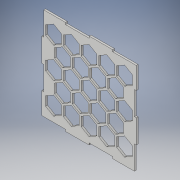
# Autodesk Inventor part: Part1
Saved by Autodesk Inventor 2019 (Build 230136000, 136)
## iProperties
Created: 2019-04-06
Part Number: Part1
Material: Generic
Document SubType Name: Modeling
Designer: Daniel
Density: 1 g/cm^3
Appearance: Default
d0: 14,549 mm
d1: 13,000 ul
d3: 28,200 mm
d4: 13,000 ul
d6: 28,200 mm
d40: 150,000 mm
d41: 150,000 mm
d42: 3,000 mm
d43: 0,00 deg
d44: 3,000 mm
d45: 37,500 mm
d46: 3,000 mm
d47: 37,500 mm
d48: 3,000 mm
d49: 37,500 mm
d50: 3,000 mm
d51: 37,500 mm
d52: 3,000 mm
d53: 37,500 mm
d54: 3,000 mm
d55: 37,500 mm
d56: 3,000 mm
d57: 3,000 mm
d58: 37,500 mm
d59: 3,000 mm
d60: 37,500 mm
d61: 37,500 mm
d62: 37,500 mm
d63: 3,000 mm
d64: 37,500 mm
d65: 3,000 mm
d66: 37,500 mm
d67: 3,000 mm
d68: 62,088 mm
d69: 0,00 deg
Author: Daniel
Autodesk Inventor part; units mm, degrees
(part 1 of 2)
ref_plane "YZ Plane" through (0, 0, 0) normal (1, 0, 0) x (0, 1, 0)
ref_plane "XZ Plane" through (0, 0, 0) normal (0, 1, 0) x (-1, 0, 0)
ref_plane "XY Plane" through (0, 0, 0) normal (0, 0, 1) x (1, 0, 0)
sketch "Sketch1" plane through (0, 0, 0) normal (0, 0, 1) x (1, 0, 0)
  line L0 (0, 0) -> (0, 14.5492)
  line L1 (0, 14.5492) -> (12.6, 7.2746)
  line L2 (12.6, 7.2746) -> (12.6, -7.2746)
  line L3 (12.6, -7.2746) -> (0, -14.5492)
  line L4 (0, -14.5492) -> (-12.6, -7.2746)
  line L5 (-12.6, -7.2746) -> (-12.6, 7.2746)
  line L6 (-12.6, 7.2746) -> (0, 14.5492)
  line L7 (0, 0) -> (-6.3, 10.9119)
  line L8 (0, 0) -> (6.4977, 11.2544)
  line L9 (-14.1, 38.9711) -> (-1.5, 31.6965)
  line L10 (-1.5, 31.6965) -> (-1.5, 17.1473)
  line L11 (-1.5, 17.1473) -> (-14.1, 9.8727)
  line L12 (-14.1, 9.8727) -> (-26.7, 17.1473)
  line L13 (-26.7, 17.1473) -> (-26.7, 31.6965)
  line L14 (-26.7, 31.6965) -> (-14.1, 38.9711)
  line L15 (-28.2, 63.3931) -> (-15.6, 56.1184)
  line L16 (-15.6, 56.1184) -> (-15.6, 41.5692)
  line L17 (-15.6, 41.5692) -> (-28.2, 34.2946)
  line L18 (-28.2, 34.2946) -> (-40.8, 41.5692)
  line L19 (-40.8, 41.5692) -> (-40.8, 56.1184)
  line L20 (-40.8, 56.1184) -> (-28.2, 63.3931)
  line L21 (-42.3, 87.815) -> (-29.7, 80.5404)
  line L22 (-29.7, 80.5404) -> (-29.7, 65.9911)
  line L23 (-29.7, 65.9911) -> (-42.3, 58.7165)
  line L24 (-42.3, 58.7165) -> (-54.9, 65.9911)
  line L25 (-54.9, 65.9911) -> (-54.9, 80.5404)
  line L26 (-54.9, 80.5404) -> (-42.3, 87.815)
  line L27 (-56.4, 112.2369) -> (-43.8, 104.9623)
  line L28 (-43.8, 104.9623) -> (-43.8, 90.4131)
  line L29 (-43.8, 90.4131) -> (-56.4, 83.1384)
  line L30 (-56.4, 83.1384) -> (-69, 90.4131)
  line L31 (-69, 90.4131) -> (-69, 104.9623)
  line L32 (-69, 104.9623) -> (-56.4, 112.2369)
  line L33 (-70.5, 136.6588) -> (-57.9, 129.3842)
  line L34 (-57.9, 129.3842) -> (-57.9, 114.835)
  line L35 (-57.9, 114.835) -> (-70.5, 107.5604)
  line L36 (-70.5, 107.5604) -> (-83.1, 114.835)
  line L37 (-83.1, 114.835) -> (-83.1, 129.3842)
  line L38 (-83.1, 129.3842) -> (-70.5, 136.6588)
  line L39 (-84.6, 161.0807) -> (-72, 153.8061)
  line L40 (-72, 153.8061) -> (-72, 139.2569)
  line L41 (-72, 139.2569) -> (-84.6, 131.9823)
  line L42 (-84.6, 131.9823) -> (-97.2, 139.2569)
  line L43 (-97.2, 139.2569) -> (-97.2, 153.8061)
  line L44 (-97.2, 153.8061) -> (-84.6, 161.0807)
  line L45 (-98.7, 185.5026) -> (-86.1, 178.228)
  line L46 (-86.1, 178.228) -> (-86.1, 163.6788)
  line L47 (-86.1, 163.6788) -> (-98.7, 156.4042)
  line L48 (-98.7, 156.4042) -> (-111.3, 163.6788)
  line L49 (-111.3, 163.6788) -> (-111.3, 178.228)
  line L50 (-111.3, 178.228) -> (-98.7, 185.5026)
  line L51 (-112.8, 209.9246) -> (-100.2, 202.6499)
  line L52 (-100.2, 202.6499) -> (-100.2, 188.1007)
  line L53 (-100.2, 188.1007) -> (-112.8, 180.8261)
  line L54 (-112.8, 180.8261) -> (-125.4, 188.1007)
  line L55 (-125.4, 188.1007) -> (-125.4, 202.6499)
  line L56 (-125.4, 202.6499) -> (-112.8, 209.9246)
  line L57 (-126.9, 234.3465) -> (-114.3, 227.0719)
  line L58 (-114.3, 227.0719) -> (-114.3, 212.5226)
  line L59 (-114.3, 212.5226) -> (-126.9, 205.248)
  line L60 (-126.9, 205.248) -> (-139.5, 212.5226)
  line L61 (-139.5, 212.5226) -> (-139.5, 227.0719)
  line L62 (-139.5, 227.0719) -> (-126.9, 234.3465)
  line L63 (-141, 258.7684) -> (-128.4, 251.4938)
  line L64 (-128.4, 251.4938) -> (-128.4, 236.9446)
  line L65 (-128.4, 236.9446) -> (-141, 229.6699)
  line L66 (-141, 229.6699) -> (-153.6, 236.9446)
  line L67 (-153.6, 236.9446) -> (-153.6, 251.4938)
  line L68 (-153.6, 251.4938) -> (-141, 258.7684)
  line L69 (-155.1, 283.1903) -> (-142.5, 275.9157)
  line L70 (-142.5, 275.9157) -> (-142.5, 261.3665)
  line L71 (-142.5, 261.3665) -> (-155.1, 254.0919)
  line L72 (-155.1, 254.0919) -> (-167.7, 261.3665)
  line L73 (-167.7, 261.3665) -> (-167.7, 275.9157)
  line L74 (-167.7, 275.9157) -> (-155.1, 283.1903)
  line L75 (-169.2, 307.6122) -> (-156.6, 300.3376)
  line L76 (-156.6, 300.3376) -> (-156.6, 285.7884)
  line L77 (-156.6, 285.7884) -> (-169.2, 278.5138)
  line L78 (-169.2, 278.5138) -> (-181.8, 285.7884)
  line L79 (-181.8, 285.7884) -> (-181.8, 300.3376)
  line L80 (-181.8, 300.3376) -> (-169.2, 307.6122)
  line L81 (14.1, 38.9711) -> (26.7, 31.6965)
  line L82 (26.7, 31.6965) -> (26.7, 17.1473)
  line L83 (26.7, 17.1473) -> (14.1, 9.8727)
  line L84 (14.1, 9.8727) -> (1.5, 17.1473)
  line L85 (1.5, 17.1473) -> (1.5, 31.6965)
  line L86 (1.5, 31.6965) -> (14.1, 38.9711)
  line L87 (0, 63.3931) -> (12.6, 56.1184)
  line L88 (12.6, 56.1184) -> (12.6, 41.5692)
  line L89 (12.6, 41.5692) -> (0, 34.2946)
  line L90 (0, 34.2946) -> (-12.6, 41.5692)
  line L91 (-12.6, 41.5692) -> (-12.6, 56.1184)
  line L92 (-12.6, 56.1184) -> (0, 63.3931)
  line L93 (-14.1, 87.815) -> (-1.5, 80.5404)
  line L94 (-1.5, 80.5404) -> (-1.5, 65.9911)
  line L95 (-1.5, 65.9911) -> (-14.1, 58.7165)
  line L96 (-14.1, 58.7165) -> (-26.7, 65.9911)
  line L97 (-26.7, 65.9911) -> (-26.7, 80.5404)
  line L98 (-26.7, 80.5404) -> (-14.1, 87.815)
  line L99 (-28.2, 112.2369) -> (-15.6, 104.9623)
  line L100 (-15.6, 104.9623) -> (-15.6, 90.4131)
  line L101 (-15.6, 90.4131) -> (-28.2, 83.1384)
  line L102 (-28.2, 83.1384) -> (-40.8, 90.4131)
  line L103 (-40.8, 90.4131) -> (-40.8, 104.9623)
  line L104 (-40.8, 104.9623) -> (-28.2, 112.2369)
  line L105 (-42.3, 136.6588) -> (-29.7, 129.3842)
  line L106 (-29.7, 129.3842) -> (-29.7, 114.835)
  line L107 (-29.7, 114.835) -> (-42.3, 107.5604)
  line L108 (-42.3, 107.5604) -> (-54.9, 114.835)
  line L109 (-54.9, 114.835) -> (-54.9, 129.3842)
  line L110 (-54.9, 129.3842) -> (-42.3, 136.6588)
  line L111 (-56.4, 161.0807) -> (-43.8, 153.8061)
  line L112 (-43.8, 153.8061) -> (-43.8, 139.2569)
  line L113 (-43.8, 139.2569) -> (-56.4, 131.9823)
  line L114 (-56.4, 131.9823) -> (-69, 139.2569)
  line L115 (-69, 139.2569) -> (-69, 153.8061)
  line L116 (-69, 153.8061) -> (-56.4, 161.0807)
  line L117 (-70.5, 185.5026) -> (-57.9, 178.228)
  line L118 (-57.9, 178.228) -> (-57.9, 163.6788)
  line L119 (-57.9, 163.6788) -> (-70.5, 156.4042)
  line L120 (-70.5, 156.4042) -> (-83.1, 163.6788)
  line L121 (-83.1, 163.6788) -> (-83.1, 178.228)
  line L122 (-83.1, 178.228) -> (-70.5, 185.5026)
  line L123 (-84.6, 209.9246) -> (-72, 202.6499)
  line L124 (-72, 202.6499) -> (-72, 188.1007)
  line L125 (-72, 188.1007) -> (-84.6, 180.8261)
  line L126 (-84.6, 180.8261) -> (-97.2, 188.1007)
  line L127 (-97.2, 188.1007) -> (-97.2, 202.6499)
  line L128 (-97.2, 202.6499) -> (-84.6, 209.9246)
  line L129 (-98.7, 234.3465) -> (-86.1, 227.0719)
  line L130 (-86.1, 227.0719) -> (-86.1, 212.5226)
  line L131 (-86.1, 212.5226) -> (-98.7, 205.248)
  line L132 (-98.7, 205.248) -> (-111.3, 212.5226)
  line L133 (-111.3, 212.5226) -> (-111.3, 227.0719)
  line L134 (-111.3, 227.0719) -> (-98.7, 234.3465)
  line L135 (-112.8, 258.7684) -> (-100.2, 251.4938)
  line L136 (-100.2, 251.4938) -> (-100.2, 236.9446)
  line L137 (-100.2, 236.9446) -> (-112.8, 229.6699)
  line L138 (-112.8, 229.6699) -> (-125.4, 236.9446)
  line L139 (-125.4, 236.9446) -> (-125.4, 251.4938)
  line L140 (-125.4, 251.4938) -> (-112.8, 258.7684)
  line L141 (-126.9, 283.1903) -> (-114.3, 275.9157)
  line L142 (-114.3, 275.9157) -> (-114.3, 261.3665)
  line L143 (-114.3, 261.3665) -> (-126.9, 254.0919)
  line L144 (-126.9, 254.0919) -> (-139.5, 261.3665)
  line L145 (-139.5, 261.3665) -> (-139.5, 275.9157)
  line L146 (-139.5, 275.9157) -> (-126.9, 283.1903)
  line L147 (-141, 307.6122) -> (-128.4, 300.3376)
  line L148 (-128.4, 300.3376) -> (-128.4, 285.7884)
  line L149 (-128.4, 285.7884) -> (-141, 278.5138)
  line L150 (-141, 278.5138) -> (-153.6, 285.7884)
  line L151 (-153.6, 285.7884) -> (-153.6, 300.3376)
  line L152 (-153.6, 300.3376) -> (-141, 307.6122)
  line L153 (-155.1, 332.0341) -> (-142.5, 324.7595)
  line L154 (-142.5, 324.7595) -> (-142.5, 310.2103)
  line L155 (-142.5, 310.2103) -> (-155.1, 302.9357)
  line L156 (-155.1, 302.9357) -> (-167.7, 310.2103)
  line L157 (-167.7, 310.2103) -> (-167.7, 324.7595)
  line L158 (-167.7, 324.7595) -> (-155.1, 332.0341)
  line L159 (28.2, 63.3931) -> (40.8, 56.1184)
  line L160 (40.8, 56.1184) -> (40.8, 41.5692)
  line L161 (40.8, 41.5692) -> (28.2, 34.2946)
  line L162 (28.2, 34.2946) -> (15.6, 41.5692)
  line L163 (15.6, 41.5692) -> (15.6, 56.1184)
  line L164 (15.6, 56.1184) -> (28.2, 63.3931)
  line L165 (14.1, 87.815) -> (26.7, 80.5404)
  line L166 (26.7, 80.5404) -> (26.7, 65.9911)
  line L167 (26.7, 65.9911) -> (14.1, 58.7165)
  line L168 (14.1, 58.7165) -> (1.5, 65.9911)
  line L169 (1.5, 65.9911) -> (1.5, 80.5404)
  line L170 (1.5, 80.5404) -> (14.1, 87.815)
  line L171 (0, 112.2369) -> (12.6, 104.9623)
  line L172 (12.6, 104.9623) -> (12.6, 90.4131)
  line L173 (12.6, 90.4131) -> (0, 83.1384)
  line L174 (0, 83.1384) -> (-12.6, 90.4131)
  line L175 (-12.6, 90.4131) -> (-12.6, 104.9623)
  line L176 (-12.6, 104.9623) -> (0, 112.2369)
  line L177 (-14.1, 136.6588) -> (-1.5, 129.3842)
  line L178 (-1.5, 129.3842) -> (-1.5, 114.835)
  line L179 (-1.5, 114.835) -> (-14.1, 107.5604)
  line L180 (-14.1, 107.5604) -> (-26.7, 114.835)
  line L181 (-26.7, 114.835) -> (-26.7, 129.3842)
  line L182 (-26.7, 129.3842) -> (-14.1, 136.6588)
  line L183 (-28.2, 161.0807) -> (-15.6, 153.8061)
  line L184 (-15.6, 153.8061) -> (-15.6, 139.2569)
  line L185 (-15.6, 139.2569) -> (-28.2, 131.9823)
  line L186 (-28.2, 131.9823) -> (-40.8, 139.2569)
  line L187 (-40.8, 139.2569) -> (-40.8, 153.8061)
  line L188 (-40.8, 153.8061) -> (-28.2, 161.0807)
  line L189 (-42.3, 185.5026) -> (-29.7, 178.228)
  line L190 (-29.7, 178.228) -> (-29.7, 163.6788)
  line L191 (-29.7, 163.6788) -> (-42.3, 156.4042)
  line L192 (-42.3, 156.4042) -> (-54.9, 163.6788)
  line L193 (-54.9, 163.6788) -> (-54.9, 178.228)
  line L194 (-54.9, 178.228) -> (-42.3, 185.5026)
  line L195 (-56.4, 209.9246) -> (-43.8, 202.6499)
  line L196 (-43.8, 202.6499) -> (-43.8, 188.1007)
  line L197 (-43.8, 188.1007) -> (-56.4, 180.8261)
  line L198 (-56.4, 180.8261) -> (-69, 188.1007)
  line L199 (-69, 188.1007) -> (-69, 202.6499)
  line L200 (-69, 202.6499) -> (-56.4, 209.9246)
  line L201 (-70.5, 234.3465) -> (-57.9, 227.0719)
  line L202 (-57.9, 227.0719) -> (-57.9, 212.5226)
  line L203 (-57.9, 212.5226) -> (-70.5, 205.248)
  line L204 (-70.5, 205.248) -> (-83.1, 212.5226)
  line L205 (-83.1, 212.5226) -> (-83.1, 227.0719)
  line L206 (-83.1, 227.0719) -> (-70.5, 234.3465)
  line L207 (-84.6, 258.7684) -> (-72, 251.4938)
  line L208 (-72, 251.4938) -> (-72, 236.9446)
  line L209 (-72, 236.9446) -> (-84.6, 229.6699)
  line L210 (-84.6, 229.6699) -> (-97.2, 236.9446)
  line L211 (-97.2, 236.9446) -> (-97.2, 251.4938)
  line L212 (-97.2, 251.4938) -> (-84.6, 258.7684)
  line L213 (-98.7, 283.1903) -> (-86.1, 275.9157)
  line L214 (-86.1, 275.9157) -> (-86.1, 261.3665)
  line L215 (-86.1, 261.3665) -> (-98.7, 254.0919)
  line L216 (-98.7, 254.0919) -> (-111.3, 261.3665)
  line L217 (-111.3, 261.3665) -> (-111.3, 275.9157)
  line L218 (-111.3, 275.9157) -> (-98.7, 283.1903)
  line L219 (-112.8, 307.6122) -> (-100.2, 300.3376)
  line L220 (-100.2, 300.3376) -> (-100.2, 285.7884)
  line L221 (-100.2, 285.7884) -> (-112.8, 278.5138)
  line L222 (-112.8, 278.5138) -> (-125.4, 285.7884)
  line L223 (-125.4, 285.7884) -> (-125.4, 300.3376)
  line L224 (-125.4, 300.3376) -> (-112.8, 307.6122)
  line L225 (-126.9, 332.0341) -> (-114.3, 324.7595)
  line L226 (-114.3, 324.7595) -> (-114.3, 310.2103)
  line L227 (-114.3, 310.2103) -> (-126.9, 302.9357)
  line L228 (-126.9, 302.9357) -> (-139.5, 310.2103)
  line L229 (-139.5, 310.2103) -> (-139.5, 324.7595)
  line L230 (-139.5, 324.7595) -> (-126.9, 332.0341)
  line L231 (-141, 356.4561) -> (-128.4, 349.1814)
  line L232 (-128.4, 349.1814) -> (-128.4, 334.6322)
  line L233 (-128.4, 334.6322) -> (-141, 327.3576)
  line L234 (-141, 327.3576) -> (-153.6, 334.6322)
  line L235 (-153.6, 334.6322) -> (-153.6, 349.1814)
  line L236 (-153.6, 349.1814) -> (-141, 356.4561)
  line L237 (42.3, 87.815) -> (54.9, 80.5404)
  line L238 (54.9, 80.5404) -> (54.9, 65.9911)
  line L239 (54.9, 65.9911) -> (42.3, 58.7165)
  line L240 (42.3, 58.7165) -> (29.7, 65.9911)
  line L241 (29.7, 65.9911) -> (29.7, 80.5404)
  line L242 (29.7, 80.5404) -> (42.3, 87.815)
  line L243 (28.2, 112.2369) -> (40.8, 104.9623)
  line L244 (40.8, 104.9623) -> (40.8, 90.4131)
  line L245 (40.8, 90.4131) -> (28.2, 83.1384)
  line L246 (28.2, 83.1384) -> (15.6, 90.4131)
  line L247 (15.6, 90.4131) -> (15.6, 104.9623)
  line L248 (15.6, 104.9623) -> (28.2, 112.2369)
  line L249 (14.1, 136.6588) -> (26.7, 129.3842)
  line L250 (26.7, 129.3842) -> (26.7, 114.835)
  line L251 (26.7, 114.835) -> (14.1, 107.5604)
  line L252 (14.1, 107.5604) -> (1.5, 114.835)
  line L253 (1.5, 114.835) -> (1.5, 129.3842)
  line L254 (1.5, 129.3842) -> (14.1, 136.6588)
  line L255 (0, 161.0807) -> (12.6, 153.8061)
  line L256 (12.6, 153.8061) -> (12.6, 139.2569)
  line L257 (12.6, 139.2569) -> (0, 131.9823)
  line L258 (0, 131.9823) -> (-12.6, 139.2569)
  line L259 (-12.6, 139.2569) -> (-12.6, 153.8061)
  line L260 (-12.6, 153.8061) -> (0, 161.0807)
  line L261 (-14.1, 185.5026) -> (-1.5, 178.228)
  line L262 (-1.5, 178.228) -> (-1.5, 163.6788)
  line L263 (-1.5, 163.6788) -> (-14.1, 156.4042)
  line L264 (-14.1, 156.4042) -> (-26.7, 163.6788)
  line L265 (-26.7, 163.6788) -> (-26.7, 178.228)
  line L266 (-26.7, 178.228) -> (-14.1, 185.5026)
  line L267 (-28.2, 209.9246) -> (-15.6, 202.6499)
  line L268 (-15.6, 202.6499) -> (-15.6, 188.1007)
  line L269 (-15.6, 188.1007) -> (-28.2, 180.8261)
  line L270 (-28.2, 180.8261) -> (-40.8, 188.1007)
  line L271 (-40.8, 188.1007) -> (-40.8, 202.6499)
  line L272 (-40.8, 202.6499) -> (-28.2, 209.9246)
  line L273 (-42.3, 234.3465) -> (-29.7, 227.0719)
  line L274 (-29.7, 227.0719) -> (-29.7, 212.5226)
  line L275 (-29.7, 212.5226) -> (-42.3, 205.248)
  line L276 (-42.3, 205.248) -> (-54.9, 212.5226)
  line L277 (-54.9, 212.5226) -> (-54.9, 227.0719)
  line L278 (-54.9, 227.0719) -> (-42.3, 234.3465)
  line L279 (-56.4, 258.7684) -> (-43.8, 251.4938)
  line L280 (-43.8, 251.4938) -> (-43.8, 236.9446)
  line L281 (-43.8, 236.9446) -> (-56.4, 229.6699)
  line L282 (-56.4, 229.6699) -> (-69, 236.9446)
  line L283 (-69, 236.9446) -> (-69, 251.4938)
  line L284 (-69, 251.4938) -> (-56.4, 258.7684)
  line L285 (-70.5, 283.1903) -> (-57.9, 275.9157)
  line L286 (-57.9, 275.9157) -> (-57.9, 261.3665)
  line L287 (-57.9, 261.3665) -> (-70.5, 254.0919)
  line L288 (-70.5, 254.0919) -> (-83.1, 261.3665)
  line L289 (-83.1, 261.3665) -> (-83.1, 275.9157)
  line L290 (-83.1, 275.9157) -> (-70.5, 283.1903)
  line L291 (-84.6, 307.6122) -> (-72, 300.3376)
  line L292 (-72, 300.3376) -> (-72, 285.7884)
  line L293 (-72, 285.7884) -> (-84.6, 278.5138)
  line L294 (-84.6, 278.5138) -> (-97.2, 285.7884)
  line L295 (-97.2, 285.7884) -> (-97.2, 300.3376)
  line L296 (-97.2, 300.3376) -> (-84.6, 307.6122)
  line L297 (-98.7, 332.0341) -> (-86.1, 324.7595)
  line L298 (-86.1, 324.7595) -> (-86.1, 310.2103)
  line L299 (-86.1, 310.2103) -> (-98.7, 302.9357)
  line L300 (-98.7, 302.9357) -> (-111.3, 310.2103)
  line L301 (-111.3, 310.2103) -> (-111.3, 324.7595)
  line L302 (-111.3, 324.7595) -> (-98.7, 332.0341)
  line L303 (-112.8, 356.4561) -> (-100.2, 349.1814)
  line L304 (-100.2, 349.1814) -> (-100.2, 334.6322)
  line L305 (-100.2, 334.6322) -> (-112.8, 327.3576)
  line L306 (-112.8, 327.3576) -> (-125.4, 334.6322)
  line L307 (-125.4, 334.6322) -> (-125.4, 349.1814)
  line L308 (-125.4, 349.1814) -> (-112.8, 356.4561)
  line L309 (-126.9, 380.878) -> (-114.3, 373.6034)
  line L310 (-114.3, 373.6034) -> (-114.3, 359.0541)
  line L311 (-114.3, 359.0541) -> (-126.9, 351.7795)
  line L312 (-126.9, 351.7795) -> (-139.5, 359.0541)
  line L313 (-139.5, 359.0541) -> (-139.5, 373.6034)
  line L314 (-139.5, 373.6034) -> (-126.9, 380.878)
  line L315 (56.4, 112.2369) -> (69, 104.9623)
  line L316 (69, 104.9623) -> (69, 90.4131)
  line L317 (69, 90.4131) -> (56.4, 83.1384)
  line L318 (56.4, 83.1384) -> (43.8, 90.4131)
  line L319 (43.8, 90.4131) -> (43.8, 104.9623)
  line L320 (43.8, 104.9623) -> (56.4, 112.2369)
  line L321 (42.3, 136.6588) -> (54.9, 129.3842)
  line L322 (54.9, 129.3842) -> (54.9, 114.835)
  line L323 (54.9, 114.835) -> (42.3, 107.5604)
  line L324 (42.3, 107.5604) -> (29.7, 114.835)
  line L325 (29.7, 114.835) -> (29.7, 129.3842)
  line L326 (29.7, 129.3842) -> (42.3, 136.6588)
  line L327 (28.2, 161.0807) -> (40.8, 153.8061)
  line L328 (40.8, 153.8061) -> (40.8, 139.2569)
  line L329 (40.8, 139.2569) -> (28.2, 131.9823)
  line L330 (28.2, 131.9823) -> (15.6, 139.2569)
  line L331 (15.6, 139.2569) -> (15.6, 153.8061)
  line L332 (15.6, 153.8061) -> (28.2, 161.0807)
  line L333 (14.1, 185.5026) -> (26.7, 178.228)
  line L334 (26.7, 178.228) -> (26.7, 163.6788)
  line L335 (26.7, 163.6788) -> (14.1, 156.4042)
  line L336 (14.1, 156.4042) -> (1.5, 163.6788)
  line L337 (1.5, 163.6788) -> (1.5, 178.228)
  line L338 (1.5, 178.228) -> (14.1, 185.5026)
  line L339 (0, 209.9246) -> (12.6, 202.6499)
  line L340 (12.6, 202.6499) -> (12.6, 188.1007)
  line L341 (12.6, 188.1007) -> (0, 180.8261)
  line L342 (0, 180.8261) -> (-12.6, 188.1007)
  line L343 (-12.6, 188.1007) -> (-12.6, 202.6499)
  line L344 (-12.6, 202.6499) -> (0, 209.9246)
  line L345 (-14.1, 234.3465) -> (-1.5, 227.0719)
  line L346 (-1.5, 227.0719) -> (-1.5, 212.5226)
  line L347 (-1.5, 212.5226) -> (-14.1, 205.248)
  line L348 (-14.1, 205.248) -> (-26.7, 212.5226)
  line L349 (-26.7, 212.5226) -> (-26.7, 227.0719)
  line L350 (-26.7, 227.0719) -> (-14.1, 234.3465)
  line L351 (-28.2, 258.7684) -> (-15.6, 251.4938)
  line L352 (-15.6, 251.4938) -> (-15.6, 236.9446)
  line L353 (-15.6, 236.9446) -> (-28.2, 229.6699)
  line L354 (-28.2, 229.6699) -> (-40.8, 236.9446)
  line L355 (-40.8, 236.9446) -> (-40.8, 251.4938)
  line L356 (-40.8, 251.4938) -> (-28.2, 258.7684)
  line L357 (-42.3, 283.1903) -> (-29.7, 275.9157)
  line L358 (-29.7, 275.9157) -> (-29.7, 261.3665)
  line L359 (-29.7, 261.3665) -> (-42.3, 254.0919)
  line L360 (-42.3, 254.0919) -> (-54.9, 261.3665)
  line L361 (-54.9, 261.3665) -> (-54.9, 275.9157)
  line L362 (-54.9, 275.9157) -> (-42.3, 283.1903)
  line L363 (-56.4, 307.6122) -> (-43.8, 300.3376)
  line L364 (-43.8, 300.3376) -> (-43.8, 285.7884)
  line L365 (-43.8, 285.7884) -> (-56.4, 278.5138)
  line L366 (-56.4, 278.5138) -> (-69, 285.7884)
  line L367 (-69, 285.7884) -> (-69, 300.3376)
  line L368 (-69, 300.3376) -> (-56.4, 307.6122)
  line L369 (-70.5, 332.0341) -> (-57.9, 324.7595)
  line L370 (-57.9, 324.7595) -> (-57.9, 310.2103)
  line L371 (-57.9, 310.2103) -> (-70.5, 302.9357)
  line L372 (-70.5, 302.9357) -> (-83.1, 310.2103)
  line L373 (-83.1, 310.2103) -> (-83.1, 324.7595)
  line L374 (-83.1, 324.7595) -> (-70.5, 332.0341)
  line L375 (-84.6, 356.4561) -> (-72, 349.1814)
  line L376 (-72, 349.1814) -> (-72, 334.6322)
  line L377 (-72, 334.6322) -> (-84.6, 327.3576)
  line L378 (-84.6, 327.3576) -> (-97.2, 334.6322)
  line L379 (-97.2, 334.6322) -> (-97.2, 349.1814)
  line L380 (-97.2, 349.1814) -> (-84.6, 356.4561)
  line L381 (-98.7, 380.878) -> (-86.1, 373.6034)
  line L382 (-86.1, 373.6034) -> (-86.1, 359.0541)
  line L383 (-86.1, 359.0541) -> (-98.7, 351.7795)
  line L384 (-98.7, 351.7795) -> (-111.3, 359.0541)
  line L385 (-111.3, 359.0541) -> (-111.3, 373.6034)
  line L386 (-111.3, 373.6034) -> (-98.7, 380.878)
  line L387 (-112.8, 405.2999) -> (-100.2, 398.0253)
  line L388 (-100.2, 398.0253) -> (-100.2, 383.476)
  line L389 (-100.2, 383.476) -> (-112.8, 376.2014)
  line L390 (-112.8, 376.2014) -> (-125.4, 383.476)
  line L391 (-125.4, 383.476) -> (-125.4, 398.0253)
  line L392 (-125.4, 398.0253) -> (-112.8, 405.2999)
  line L393 (70.5, 136.6588) -> (83.1, 129.3842)
  line L394 (83.1, 129.3842) -> (83.1, 114.835)
  line L395 (83.1, 114.835) -> (70.5, 107.5604)
  line L396 (70.5, 107.5604) -> (57.9, 114.835)
  line L397 (57.9, 114.835) -> (57.9, 129.3842)
  line L398 (57.9, 129.3842) -> (70.5, 136.6588)
  line L399 (56.4, 161.0807) -> (69, 153.8061)
  line L400 (69, 153.8061) -> (69, 139.2569)
  line L401 (69, 139.2569) -> (56.4, 131.9823)
  line L402 (56.4, 131.9823) -> (43.8, 139.2569)
  line L403 (43.8, 139.2569) -> (43.8, 153.8061)
  line L404 (43.8, 153.8061) -> (56.4, 161.0807)
  line L405 (42.3, 185.5026) -> (54.9, 178.228)
  line L406 (54.9, 178.228) -> (54.9, 163.6788)
  line L407 (54.9, 163.6788) -> (42.3, 156.4042)
  line L408 (42.3, 156.4042) -> (29.7, 163.6788)
  line L409 (29.7, 163.6788) -> (29.7, 178.228)
  line L410 (29.7, 178.228) -> (42.3, 185.5026)
  line L411 (28.2, 209.9246) -> (40.8, 202.6499)
  line L412 (40.8, 202.6499) -> (40.8, 188.1007)
  line L413 (40.8, 188.1007) -> (28.2, 180.8261)
  line L414 (28.2, 180.8261) -> (15.6, 188.1007)
  line L415 (15.6, 188.1007) -> (15.6, 202.6499)
  line L416 (15.6, 202.6499) -> (28.2, 209.9246)
  line L417 (14.1, 234.3465) -> (26.7, 227.0719)
  line L418 (26.7, 227.0719) -> (26.7, 212.5226)
  line L419 (26.7, 212.5226) -> (14.1, 205.248)
  line L420 (14.1, 205.248) -> (1.5, 212.5226)
  line L421 (1.5, 212.5226) -> (1.5, 227.0719)
  line L422 (1.5, 227.0719) -> (14.1, 234.3465)
  line L423 (0, 258.7684) -> (12.6, 251.4938)
  line L424 (12.6, 251.4938) -> (12.6, 236.9446)
  line L425 (12.6, 236.9446) -> (0, 229.6699)
  line L426 (0, 229.6699) -> (-12.6, 236.9446)
  line L427 (-12.6, 236.9446) -> (-12.6, 251.4938)
  line L428 (-12.6, 251.4938) -> (0, 258.7684)
  line L429 (-14.1, 283.1903) -> (-1.5, 275.9157)
  line L430 (-1.5, 275.9157) -> (-1.5, 261.3665)
  line L431 (-1.5, 261.3665) -> (-14.1, 254.0919)
  line L432 (-14.1, 254.0919) -> (-26.7, 261.3665)
  line L433 (-26.7, 261.3665) -> (-26.7, 275.9157)
  line L434 (-26.7, 275.9157) -> (-14.1, 283.1903)
  line L435 (-28.2, 307.6122) -> (-15.6, 300.3376)
  line L436 (-15.6, 300.3376) -> (-15.6, 285.7884)
  line L437 (-15.6, 285.7884) -> (-28.2, 278.5138)
  line L438 (-28.2, 278.5138) -> (-40.8, 285.7884)
  line L439 (-40.8, 285.7884) -> (-40.8, 300.3376)
  line L440 (-40.8, 300.3376) -> (-28.2, 307.6122)
  line L441 (-42.3, 332.0341) -> (-29.7, 324.7595)
  line L442 (-29.7, 324.7595) -> (-29.7, 310.2103)
  line L443 (-29.7, 310.2103) -> (-42.3, 302.9357)
  line L444 (-42.3, 302.9357) -> (-54.9, 310.2103)
  line L445 (-54.9, 310.2103) -> (-54.9, 324.7595)
  line L446 (-54.9, 324.7595) -> (-42.3, 332.0341)
  line L447 (-56.4, 356.4561) -> (-43.8, 349.1814)
  line L448 (-43.8, 349.1814) -> (-43.8, 334.6322)
  line L449 (-43.8, 334.6322) -> (-56.4, 327.3576)
  line L450 (-56.4, 327.3576) -> (-69, 334.6322)
  line L451 (-69, 334.6322) -> (-69, 349.1814)
  line L452 (-69, 349.1814) -> (-56.4, 356.4561)
  line L453 (-70.5, 380.878) -> (-57.9, 373.6034)
  line L454 (-57.9, 373.6034) -> (-57.9, 359.0541)
  line L455 (-57.9, 359.0541) -> (-70.5, 351.7795)
  line L456 (-70.5, 351.7795) -> (-83.1, 359.0541)
  line L457 (-83.1, 359.0541) -> (-83.1, 373.6034)
  line L458 (-83.1, 373.6034) -> (-70.5, 380.878)
  line L459 (-84.6, 405.2999) -> (-72, 398.0253)
  line L460 (-72, 398.0253) -> (-72, 383.476)
  line L461 (-72, 383.476) -> (-84.6, 376.2014)
  line L462 (-84.6, 376.2014) -> (-97.2, 383.476)
  line L463 (-97.2, 383.476) -> (-97.2, 398.0253)
  line L464 (-97.2, 398.0253) -> (-84.6, 405.2999)
  line L465 (-98.7, 429.7218) -> (-86.1, 422.4472)
  line L466 (-86.1, 422.4472) -> (-86.1, 407.898)
  line L467 (-86.1, 407.898) -> (-98.7, 400.6234)
  line L468 (-98.7, 400.6234) -> (-111.3, 407.898)
  line L469 (-111.3, 407.898) -> (-111.3, 422.4472)
  line L470 (-111.3, 422.4472) -> (-98.7, 429.7218)
  line L471 (84.6, 161.0807) -> (97.2, 153.8061)
  line L472 (97.2, 153.8061) -> (97.2, 139.2569)
  line L473 (97.2, 139.2569) -> (84.6, 131.9823)
  line L474 (84.6, 131.9823) -> (72, 139.2569)
  line L475 (72, 139.2569) -> (72, 153.8061)
  line L476 (72, 153.8061) -> (84.6, 161.0807)
  line L477 (70.5, 185.5026) -> (83.1, 178.228)
  line L478 (83.1, 178.228) -> (83.1, 163.6788)
  line L479 (83.1, 163.6788) -> (70.5, 156.4042)
  line L480 (70.5, 156.4042) -> (57.9, 163.6788)
  line L481 (57.9, 163.6788) -> (57.9, 178.228)
  line L482 (57.9, 178.228) -> (70.5, 185.5026)
  line L483 (56.4, 209.9246) -> (69, 202.6499)
  line L484 (69, 202.6499) -> (69, 188.1007)
  line L485 (69, 188.1007) -> (56.4, 180.8261)
  line L486 (56.4, 180.8261) -> (43.8, 188.1007)
  line L487 (43.8, 188.1007) -> (43.8, 202.6499)
  line L488 (43.8, 202.6499) -> (56.4, 209.9246)
  line L489 (42.3, 234.3465) -> (54.9, 227.0719)
  line L490 (54.9, 227.0719) -> (54.9, 212.5226)
  line L491 (54.9, 212.5226) -> (42.3, 205.248)
  line L492 (42.3, 205.248) -> (29.7, 212.5226)
  line L493 (29.7, 212.5226) -> (29.7, 227.0719)
  line L494 (29.7, 227.0719) -> (42.3, 234.3465)
  line L495 (28.2, 258.7684) -> (40.8, 251.4938)
  line L496 (40.8, 251.4938) -> (40.8, 236.9446)
  line L497 (40.8, 236.9446) -> (28.2, 229.6699)
  line L498 (28.2, 229.6699) -> (15.6, 236.9446)
  line L499 (15.6, 236.9446) -> (15.6, 251.4938)
  line L500 (15.6, 251.4938) -> (28.2, 258.7684)
  line L501 (14.1, 283.1903) -> (26.7, 275.9157)
  line L502 (26.7, 275.9157) -> (26.7, 261.3665)
  line L503 (26.7, 261.3665) -> (14.1, 254.0919)
  line L504 (14.1, 254.0919) -> (1.5, 261.3665)
  line L505 (1.5, 261.3665) -> (1.5, 275.9157)
  line L506 (1.5, 275.9157) -> (14.1, 283.1903)
  line L507 (0, 307.6122) -> (12.6, 300.3376)
  line L508 (12.6, 300.3376) -> (12.6, 285.7884)
  line L509 (12.6, 285.7884) -> (0, 278.5138)
  line L510 (0, 278.5138) -> (-12.6, 285.7884)
  line L511 (-12.6, 285.7884) -> (-12.6, 300.3376)
  line L512 (-12.6, 300.3376) -> (0, 307.6122)
  line L513 (-14.1, 332.0341) -> (-1.5, 324.7595)
  line L514 (-1.5, 324.7595) -> (-1.5, 310.2103)
  line L515 (-1.5, 310.2103) -> (-14.1, 302.9357)
  line L516 (-14.1, 302.9357) -> (-26.7, 310.2103)
  line L517 (-26.7, 310.2103) -> (-26.7, 324.7595)
  line L518 (-26.7, 324.7595) -> (-14.1, 332.0341)
  line L519 (-28.2, 356.4561) -> (-15.6, 349.1814)
  line L520 (-15.6, 349.1814) -> (-15.6, 334.6322)
  line L521 (-15.6, 334.6322) -> (-28.2, 327.3576)
  line L522 (-28.2, 327.3576) -> (-40.8, 334.6322)
  line L523 (-40.8, 334.6322) -> (-40.8, 349.1814)
  line L524 (-40.8, 349.1814) -> (-28.2, 356.4561)
  line L525 (-42.3, 380.878) -> (-29.7, 373.6034)
  line L526 (-29.7, 373.6034) -> (-29.7, 359.0541)
  line L527 (-29.7, 359.0541) -> (-42.3, 351.7795)
  line L528 (-42.3, 351.7795) -> (-54.9, 359.0541)
  line L529 (-54.9, 359.0541) -> (-54.9, 373.6034)
  line L530 (-54.9, 373.6034) -> (-42.3, 380.878)
  line L531 (-56.4, 405.2999) -> (-43.8, 398.0253)
  line L532 (-43.8, 398.0253) -> (-43.8, 383.476)
  line L533 (-43.8, 383.476) -> (-56.4, 376.2014)
  line L534 (-56.4, 376.2014) -> (-69, 383.476)
  line L535 (-69, 383.476) -> (-69, 398.0253)
  line L536 (-69, 398.0253) -> (-56.4, 405.2999)
  line L537 (-70.5, 429.7218) -> (-57.9, 422.4472)
  line L538 (-57.9, 422.4472) -> (-57.9, 407.898)
  line L539 (-57.9, 407.898) -> (-70.5, 400.6234)
  line L540 (-70.5, 400.6234) -> (-83.1, 407.898)
  line L541 (-83.1, 407.898) -> (-83.1, 422.4472)
  line L542 (-83.1, 422.4472) -> (-70.5, 429.7218)
  line L543 (-84.6, 454.1437) -> (-72, 446.8691)
  line L544 (-72, 446.8691) -> (-72, 432.3199)
  line L545 (-72, 432.3199) -> (-84.6, 425.0453)
  line L546 (-84.6, 425.0453) -> (-97.2, 432.3199)
  line L547 (-97.2, 432.3199) -> (-97.2, 446.8691)
  line L548 (-97.2, 446.8691) -> (-84.6, 454.1437)
  line L549 (98.7, 185.5026) -> (111.3, 178.228)
  line L550 (111.3, 178.228) -> (111.3, 163.6788)
  line L551 (111.3, 163.6788) -> (98.7, 156.4042)
  line L552 (98.7, 156.4042) -> (86.1, 163.6788)
  line L553 (86.1, 163.6788) -> (86.1, 178.228)
  line L554 (86.1, 178.228) -> (98.7, 185.5026)
  line L555 (84.6, 209.9246) -> (97.2, 202.6499)
  line L556 (97.2, 202.6499) -> (97.2, 188.1007)
  line L557 (97.2, 188.1007) -> (84.6, 180.8261)
  line L558 (84.6, 180.8261) -> (72, 188.1007)
  line L559 (72, 188.1007) -> (72, 202.6499)
  line L560 (72, 202.6499) -> (84.6, 209.9246)
  line L561 (70.5, 234.3465) -> (83.1, 227.0719)
  line L562 (83.1, 227.0719) -> (83.1, 212.5226)
  line L563 (83.1, 212.5226) -> (70.5, 205.248)
  line L564 (70.5, 205.248) -> (57.9, 212.5226)
  line L565 (57.9, 212.5226) -> (57.9, 227.0719)
  line L566 (57.9, 227.0719) -> (70.5, 234.3465)
  line L567 (56.4, 258.7684) -> (69, 251.4938)
  line L568 (69, 251.4938) -> (69, 236.9446)
  line L569 (69, 236.9446) -> (56.4, 229.6699)
  line L570 (56.4, 229.6699) -> (43.8, 236.9446)
  line L571 (43.8, 236.9446) -> (43.8, 251.4938)
  line L572 (43.8, 251.4938) -> (56.4, 258.7684)
  line L573 (42.3, 283.1903) -> (54.9, 275.9157)
  line L574 (54.9, 275.9157) -> (54.9, 261.3665)
  line L575 (54.9, 261.3665) -> (42.3, 254.0919)
  line L576 (42.3, 254.0919) -> (29.7, 261.3665)
  line L577 (29.7, 261.3665) -> (29.7, 275.9157)
  line L578 (29.7, 275.9157) -> (42.3, 283.1903)
  line L579 (28.2, 307.6122) -> (40.8, 300.3376)
  line L580 (40.8, 300.3376) -> (40.8, 285.7884)
  line L581 (40.8, 285.7884) -> (28.2, 278.5138)
  line L582 (28.2, 278.5138) -> (15.6, 285.7884)
  line L583 (15.6, 285.7884) -> (15.6, 300.3376)
  line L584 (15.6, 300.3376) -> (28.2, 307.6122)
  line L585 (14.1, 332.0341) -> (26.7, 324.7595)
  line L586 (26.7, 324.7595) -> (26.7, 310.2103)
  line L587 (26.7, 310.2103) -> (14.1, 302.9357)
  line L588 (14.1, 302.9357) -> (1.5, 310.2103)
  line L589 (1.5, 310.2103) -> (1.5, 324.7595)
  line L590 (1.5, 324.7595) -> (14.1, 332.0341)
  line L591 (0, 356.4561) -> (12.6, 349.1814)
  line L592 (12.6, 349.1814) -> (12.6, 334.6322)
  line L593 (12.6, 334.6322) -> (0, 327.3576)
  line L594 (0, 327.3576) -> (-12.6, 334.6322)
  line L595 (-12.6, 334.6322) -> (-12.6, 349.1814)
  line L596 (-12.6, 349.1814) -> (0, 356.4561)
  line L597 (-14.1, 380.878) -> (-1.5, 373.6034)
  line L598 (-1.5, 373.6034) -> (-1.5, 359.0541)
  line L599 (-1.5, 359.0541) -> (-14.1, 351.7795)
  line L600 (-14.1, 351.7795) -> (-26.7, 359.0541)
  line L601 (-26.7, 359.0541) -> (-26.7, 373.6034)
  line L602 (-26.7, 373.6034) -> (-14.1, 380.878)
  line L603 (-28.2, 405.2999) -> (-15.6, 398.0253)
  line L604 (-15.6, 398.0253) -> (-15.6, 383.476)
  line L605 (-15.6, 383.476) -> (-28.2, 376.2014)
  line L606 (-28.2, 376.2014) -> (-40.8, 383.476)
  line L607 (-40.8, 383.476) -> (-40.8, 398.0253)
  line L608 (-40.8, 398.0253) -> (-28.2, 405.2999)
  line L609 (-42.3, 429.7218) -> (-29.7, 422.4472)
  line L610 (-29.7, 422.4472) -> (-29.7, 407.898)
  line L611 (-29.7, 407.898) -> (-42.3, 400.6234)
  line L612 (-42.3, 400.6234) -> (-54.9, 407.898)
  line L613 (-54.9, 407.898) -> (-54.9, 422.4472)
  line L614 (-54.9, 422.4472) -> (-42.3, 429.7218)
  line L615 (-56.4, 454.1437) -> (-43.8, 446.8691)
  line L616 (-43.8, 446.8691) -> (-43.8, 432.3199)
  line L617 (-43.8, 432.3199) -> (-56.4, 425.0453)
  line L618 (-56.4, 425.0453) -> (-69, 432.3199)
  line L619 (-69, 432.3199) -> (-69, 446.8691)
  line L620 (-69, 446.8691) -> (-56.4, 454.1437)
  line L621 (-70.5, 478.5656) -> (-57.9, 471.291)
  line L622 (-57.9, 471.291) -> (-57.9, 456.7418)
  line L623 (-57.9, 456.7418) -> (-70.5, 449.4672)
  line L624 (-70.5, 449.4672) -> (-83.1, 456.7418)
  line L625 (-83.1, 456.7418) -> (-83.1, 471.291)
  line L626 (-83.1, 471.291) -> (-70.5, 478.5656)
  line L627 (112.8, 209.9246) -> (125.4, 202.6499)
  line L628 (125.4, 202.6499) -> (125.4, 188.1007)
  line L629 (125.4, 188.1007) -> (112.8, 180.8261)
  line L630 (112.8, 180.8261) -> (100.2, 188.1007)
  line L631 (100.2, 188.1007) -> (100.2, 202.6499)
  line L632 (100.2, 202.6499) -> (112.8, 209.9246)
  line L633 (98.7, 234.3465) -> (111.3, 227.0719)
  line L634 (111.3, 227.0719) -> (111.3, 212.5226)
  line L635 (111.3, 212.5226) -> (98.7, 205.248)
  line L636 (98.7, 205.248) -> (86.1, 212.5226)
  line L637 (86.1, 212.5226) -> (86.1, 227.0719)
  line L638 (86.1, 227.0719) -> (98.7, 234.3465)
  line L639 (84.6, 258.7684) -> (97.2, 251.4938)
  line L640 (97.2, 251.4938) -> (97.2, 236.9446)
  line L641 (97.2, 236.9446) -> (84.6, 229.6699)
  line L642 (84.6, 229.6699) -> (72, 236.9446)
  line L643 (72, 236.9446) -> (72, 251.4938)
  line L644 (72, 251.4938) -> (84.6, 258.7684)
  line L645 (70.5, 283.1903) -> (83.1, 275.9157)
  line L646 (83.1, 275.9157) -> (83.1, 261.3665)
  line L647 (83.1, 261.3665) -> (70.5, 254.0919)
  line L648 (70.5, 254.0919) -> (57.9, 261.3665)
  line L649 (57.9, 261.3665) -> (57.9, 275.9157)
  line L650 (57.9, 275.9157) -> (70.5, 283.1903)
  line L651 (56.4, 307.6122) -> (69, 300.3376)
  line L652 (69, 300.3376) -> (69, 285.7884)
  line L653 (69, 285.7884) -> (56.4, 278.5138)
  line L654 (56.4, 278.5138) -> (43.8, 285.7884)
  line L655 (43.8, 285.7884) -> (43.8, 300.3376)
  line L656 (43.8, 300.3376) -> (56.4, 307.6122)
  line L657 (42.3, 332.0341) -> (54.9, 324.7595)
  line L658 (54.9, 324.7595) -> (54.9, 310.2103)
  line L659 (54.9, 310.2103) -> (42.3, 302.9357)
  line L660 (42.3, 302.9357) -> (29.7, 310.2103)
  line L661 (29.7, 310.2103) -> (29.7, 324.7595)
  line L662 (29.7, 324.7595) -> (42.3, 332.0341)
  line L663 (28.2, 356.4561) -> (40.8, 349.1814)
  line L664 (40.8, 349.1814) -> (40.8, 334.6322)
  line L665 (40.8, 334.6322) -> (28.2, 327.3576)
  line L666 (28.2, 327.3576) -> (15.6, 334.6322)
  line L667 (15.6, 334.6322) -> (15.6, 349.1814)
  line L668 (15.6, 349.1814) -> (28.2, 356.4561)
  line L669 (14.1, 380.878) -> (26.7, 373.6034)
  line L670 (26.7, 373.6034) -> (26.7, 359.0541)
  line L671 (26.7, 359.0541) -> (14.1, 351.7795)
  line L672 (14.1, 351.7795) -> (1.5, 359.0541)
  line L673 (1.5, 359.0541) -> (1.5, 373.6034)
  line L674 (1.5, 373.6034) -> (14.1, 380.878)
  line L675 (0, 405.2999) -> (12.6, 398.0253)
  line L676 (12.6, 398.0253) -> (12.6, 383.476)
  line L677 (12.6, 383.476) -> (0, 376.2014)
  line L678 (0, 376.2014) -> (-12.6, 383.476)
  line L679 (-12.6, 383.476) -> (-12.6, 398.0253)
  line L680 (-12.6, 398.0253) -> (0, 405.2999)
  line L681 (-14.1, 429.7218) -> (-1.5, 422.4472)
  line L682 (-1.5, 422.4472) -> (-1.5, 407.898)
  line L683 (-1.5, 407.898) -> (-14.1, 400.6234)
  line L684 (-14.1, 400.6234) -> (-26.7, 407.898)
  line L685 (-26.7, 407.898) -> (-26.7, 422.4472)
  line L686 (-26.7, 422.4472) -> (-14.1, 429.7218)
  line L687 (-28.2, 454.1437) -> (-15.6, 446.8691)
  line L688 (-15.6, 446.8691) -> (-15.6, 432.3199)
  line L689 (-15.6, 432.3199) -> (-28.2, 425.0453)
  line L690 (-28.2, 425.0453) -> (-40.8, 432.3199)
  line L691 (-40.8, 432.3199) -> (-40.8, 446.8691)
  line L692 (-40.8, 446.8691) -> (-28.2, 454.1437)
  line L693 (-42.3, 478.5656) -> (-29.7, 471.291)
  line L694 (-29.7, 471.291) -> (-29.7, 456.7418)
  line L695 (-29.7, 456.7418) -> (-42.3, 449.4672)
  line L696 (-42.3, 449.4672) -> (-54.9, 456.7418)
  line L697 (-54.9, 456.7418) -> (-54.9, 471.291)
  line L698 (-54.9, 471.291) -> (-42.3, 478.5656)
  line L699 (-56.4, 502.9876) -> (-43.8, 495.7129)
  line L700 (-43.8, 495.7129) -> (-43.8, 481.1637)
  line L701 (-43.8, 481.1637) -> (-56.4, 473.8891)
  line L702 (-56.4, 473.8891) -> (-69, 481.1637)
  line L703 (-69, 481.1637) -> (-69, 495.7129)
  line L704 (-69, 495.7129) -> (-56.4, 502.9876)
  line L705 (126.9, 234.3465) -> (139.5, 227.0719)
  line L706 (139.5, 227.0719) -> (139.5, 212.5226)
  line L707 (139.5, 212.5226) -> (126.9, 205.248)
  line L708 (126.9, 205.248) -> (114.3, 212.5226)
  line L709 (114.3, 212.5226) -> (114.3, 227.0719)
  line L710 (114.3, 227.0719) -> (126.9, 234.3465)
  line L711 (112.8, 258.7684) -> (125.4, 251.4938)
  line L712 (125.4, 251.4938) -> (125.4, 236.9446)
  line L713 (125.4, 236.9446) -> (112.8, 229.6699)
  line L714 (112.8, 229.6699) -> (100.2, 236.9446)
  line L715 (100.2, 236.9446) -> (100.2, 251.4938)
  line L716 (100.2, 251.4938) -> (112.8, 258.7684)
  line L717 (98.7, 283.1903) -> (111.3, 275.9157)
  line L718 (111.3, 275.9157) -> (111.3, 261.3665)
  line L719 (111.3, 261.3665) -> (98.7, 254.0919)
  line L720 (98.7, 254.0919) -> (86.1, 261.3665)
  line L721 (86.1, 261.3665) -> (86.1, 275.9157)
  line L722 (86.1, 275.9157) -> (98.7, 283.1903)
  line L723 (84.6, 307.6122) -> (97.2, 300.3376)
  line L724 (97.2, 300.3376) -> (97.2, 285.7884)
  line L725 (97.2, 285.7884) -> (84.6, 278.5138)
  line L726 (84.6, 278.5138) -> (72, 285.7884)
  line L727 (72, 285.7884) -> (72, 300.3376)
  line L728 (72, 300.3376) -> (84.6, 307.6122)
  line L729 (70.5, 332.0341) -> (83.1, 324.7595)
  line L730 (83.1, 324.7595) -> (83.1, 310.2103)
  line L731 (83.1, 310.2103) -> (70.5, 302.9357)
  line L732 (70.5, 302.9357) -> (57.9, 310.2103)
  line L733 (57.9, 310.2103) -> (57.9, 324.7595)
  line L734 (57.9, 324.7595) -> (70.5, 332.0341)
  line L735 (56.4, 356.4561) -> (69, 349.1814)
  line L736 (69, 349.1814) -> (69, 334.6322)
  line L737 (69, 334.6322) -> (56.4, 327.3576)
  line L738 (56.4, 327.3576) -> (43.8, 334.6322)
  line L739 (43.8, 334.6322) -> (43.8, 349.1814)
  line L740 (43.8, 349.1814) -> (56.4, 356.4561)
  line L741 (42.3, 380.878) -> (54.9, 373.6034)
  line L742 (54.9, 373.6034) -> (54.9, 359.0541)
  line L743 (54.9, 359.0541) -> (42.3, 351.7795)
  line L744 (42.3, 351.7795) -> (29.7, 359.0541)
  line L745 (29.7, 359.0541) -> (29.7, 373.6034)
  line L746 (29.7, 373.6034) -> (42.3, 380.878)
  line L747 (28.2, 405.2999) -> (40.8, 398.0253)
  line L748 (40.8, 398.0253) -> (40.8, 383.476)
  line L749 (40.8, 383.476) -> (28.2, 376.2014)
  line L750 (28.2, 376.2014) -> (15.6, 383.476)
  line L751 (15.6, 383.476) -> (15.6, 398.0253)
  line L752 (15.6, 398.0253) -> (28.2, 405.2999)
  line L753 (14.1, 429.7218) -> (26.7, 422.4472)
  line L754 (26.7, 422.4472) -> (26.7, 407.898)
  line L755 (26.7, 407.898) -> (14.1, 400.6234)
  line L756 (14.1, 400.6234) -> (1.5, 407.898)
  line L757 (1.5, 407.898) -> (1.5, 422.4472)
  line L758 (1.5, 422.4472) -> (14.1, 429.7218)
  line L759 (0, 454.1437) -> (12.6, 446.8691)
  line L760 (12.6, 446.8691) -> (12.6, 432.3199)
  line L761 (12.6, 432.3199) -> (0, 425.0453)
  line L762 (0, 425.0453) -> (-12.6, 432.3199)
  line L763 (-12.6, 432.3199) -> (-12.6, 446.8691)
  line L764 (-12.6, 446.8691) -> (0, 454.1437)
  line L765 (-14.1, 478.5656) -> (-1.5, 471.291)
  line L766 (-1.5, 471.291) -> (-1.5, 456.7418)
  line L767 (-1.5, 456.7418) -> (-14.1, 449.4672)
  line L768 (-14.1, 449.4672) -> (-26.7, 456.7418)
  line L769 (-26.7, 456.7418) -> (-26.7, 471.291)
  line L770 (-26.7, 471.291) -> (-14.1, 478.5656)
  line L771 (-28.2, 502.9876) -> (-15.6, 495.7129)
  line L772 (-15.6, 495.7129) -> (-15.6, 481.1637)
  line L773 (-15.6, 481.1637) -> (-28.2, 473.8891)
  line L774 (-28.2, 473.8891) -> (-40.8, 481.1637)
  line L775 (-40.8, 481.1637) -> (-40.8, 495.7129)
  line L776 (-40.8, 495.7129) -> (-28.2, 502.9876)
  line L777 (-42.3, 527.4095) -> (-29.7, 520.1349)
  line L778 (-29.7, 520.1349) -> (-29.7, 505.5856)
  line L779 (-29.7, 505.5856) -> (-42.3, 498.311)
  line L780 (-42.3, 498.311) -> (-54.9, 505.5856)
  line L781 (-54.9, 505.5856) -> (-54.9, 520.1349)
  line L782 (-54.9, 520.1349) -> (-42.3, 527.4095)
  line L783 (141, 258.7684) -> (153.6, 251.4938)
  line L784 (153.6, 251.4938) -> (153.6, 236.9446)
  line L785 (153.6, 236.9446) -> (141, 229.6699)
  line L786 (141, 229.6699) -> (128.4, 236.9446)
  line L787 (128.4, 236.9446) -> (128.4, 251.4938)
  line L788 (128.4, 251.4938) -> (141, 258.7684)
  line L789 (126.9, 283.1903) -> (139.5, 275.9157)
  line L790 (139.5, 275.9157) -> (139.5, 261.3665)
  line L791 (139.5, 261.3665) -> (126.9, 254.0919)
  line L792 (126.9, 254.0919) -> (114.3, 261.3665)
  line L793 (114.3, 261.3665) -> (114.3, 275.9157)
  line L794 (114.3, 275.9157) -> (126.9, 283.1903)
  line L795 (112.8, 307.6122) -> (125.4, 300.3376)
  line L796 (125.4, 300.3376) -> (125.4, 285.7884)
  line L797 (125.4, 285.7884) -> (112.8, 278.5138)
  line L798 (112.8, 278.5138) -> (100.2, 285.7884)
  line L799 (100.2, 285.7884) -> (100.2, 300.3376)
  line L800 (100.2, 300.3376) -> (112.8, 307.6122)
  line L801 (98.7, 332.0341) -> (111.3, 324.7595)
  line L802 (111.3, 324.7595) -> (111.3, 310.2103)
  line L803 (111.3, 310.2103) -> (98.7, 302.9357)
  line L804 (98.7, 302.9357) -> (86.1, 310.2103)
  line L805 (86.1, 310.2103) -> (86.1, 324.7595)
  line L806 (86.1, 324.7595) -> (98.7, 332.0341)
  line L807 (84.6, 356.4561) -> (97.2, 349.1814)
  line L808 (97.2, 349.1814) -> (97.2, 334.6322)
  line L809 (97.2, 334.6322) -> (84.6, 327.3576)
  line L810 (84.6, 327.3576) -> (72, 334.6322)
  line L811 (72, 334.6322) -> (72, 349.1814)
  line L812 (72, 349.1814) -> (84.6, 356.4561)
  line L813 (70.5, 380.878) -> (83.1, 373.6034)
  line L814 (83.1, 373.6034) -> (83.1, 359.0541)
  line L815 (83.1, 359.0541) -> (70.5, 351.7795)
  line L816 (70.5, 351.7795) -> (57.9, 359.0541)
  line L817 (57.9, 359.0541) -> (57.9, 373.6034)
  line L818 (57.9, 373.6034) -> (70.5, 380.878)
  line L819 (56.4, 405.2999) -> (69, 398.0253)
  line L820 (69, 398.0253) -> (69, 383.476)
  line L821 (69, 383.476) -> (56.4, 376.2014)
  line L822 (56.4, 376.2014) -> (43.8, 383.476)
  line L823 (43.8, 383.476) -> (43.8, 398.0253)
  line L824 (43.8, 398.0253) -> (56.4, 405.2999)
  line L825 (42.3, 429.7218) -> (54.9, 422.4472)
  line L826 (54.9, 422.4472) -> (54.9, 407.898)
  line L827 (54.9, 407.898) -> (42.3, 400.6234)
  line L828 (42.3, 400.6234) -> (29.7, 407.898)
  line L829 (29.7, 407.898) -> (29.7, 422.4472)
  line L830 (29.7, 422.4472) -> (42.3, 429.7218)
  line L831 (28.2, 454.1437) -> (40.8, 446.8691)
  line L832 (40.8, 446.8691) -> (40.8, 432.3199)
  line L833 (40.8, 432.3199) -> (28.2, 425.0453)
  line L834 (28.2, 425.0453) -> (15.6, 432.3199)
  line L835 (15.6, 432.3199) -> (15.6, 446.8691)
  line L836 (15.6, 446.8691) -> (28.2, 454.1437)
  line L837 (14.1, 478.5656) -> (26.7, 471.291)
  line L838 (26.7, 471.291) -> (26.7, 456.7418)
  line L839 (26.7, 456.7418) -> (14.1, 449.4672)
  line L840 (14.1, 449.4672) -> (1.5, 456.7418)
  line L841 (1.5, 456.7418) -> (1.5, 471.291)
  line L842 (1.5, 471.291) -> (14.1, 478.5656)
  line L843 (0, 502.9876) -> (12.6, 495.7129)
  line L844 (12.6, 495.7129) -> (12.6, 481.1637)
  line L845 (12.6, 481.1637) -> (0, 473.8891)
  line L846 (0, 473.8891) -> (-12.6, 481.1637)
  line L847 (-12.6, 481.1637) -> (-12.6, 495.7129)
  line L848 (-12.6, 495.7129) -> (0, 502.9876)
  line L849 (-14.1, 527.4095) -> (-1.5, 520.1349)
  line L850 (-1.5, 520.1349) -> (-1.5, 505.5856)
  line L851 (-1.5, 505.5856) -> (-14.1, 498.311)
  line L852 (-14.1, 498.311) -> (-26.7, 505.5856)
  line L853 (-26.7, 505.5856) -> (-26.7, 520.1349)
  line L854 (-26.7, 520.1349) -> (-14.1, 527.4095)
  line L855 (-28.2, 551.8314) -> (-15.6, 544.5568)
  line L856 (-15.6, 544.5568) -> (-15.6, 530.0075)
  line L857 (-15.6, 530.0075) -> (-28.2, 522.7329)
  line L858 (-28.2, 522.7329) -> (-40.8, 530.0075)
  line L859 (-40.8, 530.0075) -> (-40.8, 544.5568)
  line L860 (-40.8, 544.5568) -> (-28.2, 551.8314)
  line L861 (155.1, 283.1903) -> (167.7, 275.9157)
  line L862 (167.7, 275.9157) -> (167.7, 261.3665)
  line L863 (167.7, 261.3665) -> (155.1, 254.0919)
  line L864 (155.1, 254.0919) -> (142.5, 261.3665)
  line L865 (142.5, 261.3665) -> (142.5, 275.9157)
  line L866 (142.5, 275.9157) -> (155.1, 283.1903)
  line L867 (141, 307.6122) -> (153.6, 300.3376)
  line L868 (153.6, 300.3376) -> (153.6, 285.7884)
  line L869 (153.6, 285.7884) -> (141, 278.5138)
  line L870 (141, 278.5138) -> (128.4, 285.7884)
  line L871 (128.4, 285.7884) -> (128.4, 300.3376)
  line L872 (128.4, 300.3376) -> (141, 307.6122)
  line L873 (126.9, 332.0341) -> (139.5, 324.7595)
  line L874 (139.5, 324.7595) -> (139.5, 310.2103)
  line L875 (139.5, 310.2103) -> (126.9, 302.9357)
  line L876 (126.9, 302.9357) -> (114.3, 310.2103)
  line L877 (114.3, 310.2103) -> (114.3, 324.7595)
  line L878 (114.3, 324.7595) -> (126.9, 332.0341)
  line L879 (112.8, 356.4561) -> (125.4, 349.1814)
  line L880 (125.4, 349.1814) -> (125.4, 334.6322)
  line L881 (125.4, 334.6322) -> (112.8, 327.3576)
  line L882 (112.8, 327.3576) -> (100.2, 334.6322)
  line L883 (100.2, 334.6322) -> (100.2, 349.1814)
  line L884 (100.2, 349.1814) -> (112.8, 356.4561)
  line L885 (98.7, 380.878) -> (111.3, 373.6034)
  line L886 (111.3, 373.6034) -> (111.3, 359.0541)
  line L887 (111.3, 359.0541) -> (98.7, 351.7795)
  line L888 (98.7, 351.7795) -> (86.1, 359.0541)
  line L889 (86.1, 359.0541) -> (86.1, 373.6034)
  line L890 (86.1, 373.6034) -> (98.7, 380.878)
  line L891 (84.6, 405.2999) -> (97.2, 398.0253)
  line L892 (97.2, 398.0253) -> (97.2, 383.476)
  line L893 (97.2, 383.476) -> (84.6, 376.2014)
  line L894 (84.6, 376.2014) -> (72, 383.476)
  line L895 (72, 383.476) -> (72, 398.0253)
  line L896 (72, 398.0253) -> (84.6, 405.2999)
  line L897 (70.5, 429.7218) -> (83.1, 422.4472)
  line L898 (83.1, 422.4472) -> (83.1, 407.898)
  line L899 (83.1, 407.898) -> (70.5, 400.6234)
  line L900 (70.5, 400.6234) -> (57.9, 407.898)
  line L901 (57.9, 407.898) -> (57.9, 422.4472)
  line L902 (57.9, 422.4472) -> (70.5, 429.7218)
  line L903 (56.4, 454.1437) -> (69, 446.8691)
  line L904 (69, 446.8691) -> (69, 432.3199)
  line L905 (69, 432.3199) -> (56.4, 425.0453)
  line L906 (56.4, 425.0453) -> (43.8, 432.3199)
  line L907 (43.8, 432.3199) -> (43.8, 446.8691)
  line L908 (43.8, 446.8691) -> (56.4, 454.1437)
  line L909 (42.3, 478.5656) -> (54.9, 471.291)
  line L910 (54.9, 471.291) -> (54.9, 456.7418)
  line L911 (54.9, 456.7418) -> (42.3, 449.4672)
  line L912 (42.3, 449.4672) -> (29.7, 456.7418)
  line L913 (29.7, 456.7418) -> (29.7, 471.291)
  line L914 (29.7, 471.291) -> (42.3, 478.5656)
  line L915 (28.2, 502.9876) -> (40.8, 495.7129)
  line L916 (40.8, 495.7129) -> (40.8, 481.1637)
  line L917 (40.8, 481.1637) -> (28.2, 473.8891)
  line L918 (28.2, 473.8891) -> (15.6, 481.1637)
  line L919 (15.6, 481.1637) -> (15.6, 495.7129)
  line L920 (15.6, 495.7129) -> (28.2, 502.9876)
  line L921 (14.1, 527.4095) -> (26.7, 520.1349)
  line L922 (26.7, 520.1349) -> (26.7, 505.5856)
  line L923 (26.7, 505.5856) -> (14.1, 498.311)
  line L924 (14.1, 498.311) -> (1.5, 505.5856)
  line L925 (1.5, 505.5856) -> (1.5, 520.1349)
  line L926 (1.5, 520.1349) -> (14.1, 527.4095)
  line L927 (0, 551.8314) -> (12.6, 544.5568)
  line L928 (12.6, 544.5568) -> (12.6, 530.0075)
  line L929 (12.6, 530.0075) -> (0, 522.7329)
  line L930 (0, 522.7329) -> (-12.6, 530.0075)
  line L931 (-12.6, 530.0075) -> (-12.6, 544.5568)
  line L932 (-12.6, 544.5568) -> (0, 551.8314)
  line L933 (-14.1, 576.2533) -> (-1.5, 568.9787)
  line L934 (-1.5, 568.9787) -> (-1.5, 554.4295)
  line L935 (-1.5, 554.4295) -> (-14.1, 547.1549)
  line L936 (-14.1, 547.1549) -> (-26.7, 554.4295)
  line L937 (-26.7, 554.4295) -> (-26.7, 568.9787)
  line L938 (-26.7, 568.9787) -> (-14.1, 576.2533)
  line L939 (169.2, 307.6122) -> (181.8, 300.3376)
  line L940 (181.8, 300.3376) -> (181.8, 285.7884)
  line L941 (181.8, 285.7884) -> (169.2, 278.5138)
  line L942 (169.2, 278.5138) -> (156.6, 285.7884)
  line L943 (156.6, 285.7884) -> (156.6, 300.3376)
  line L944 (156.6, 300.3376) -> (169.2, 307.6122)
  line L945 (155.1, 332.0341) -> (167.7, 324.7595)
  line L946 (167.7, 324.7595) -> (167.7, 310.2103)
  line L947 (167.7, 310.2103) -> (155.1, 302.9357)
  line L948 (155.1, 302.9357) -> (142.5, 310.2103)
  line L949 (142.5, 310.2103) -> (142.5, 324.7595)
  line L950 (142.5, 324.7595) -> (155.1, 332.0341)
  line L951 (141, 356.4561) -> (153.6, 349.1814)
  line L952 (153.6, 349.1814) -> (153.6, 334.6322)
  line L953 (153.6, 334.6322) -> (141, 327.3576)
  line L954 (141, 327.3576) -> (128.4, 334.6322)
  line L955 (128.4, 334.6322) -> (128.4, 349.1814)
  line L956 (128.4, 349.1814) -> (141, 356.4561)
  line L957 (126.9, 380.878) -> (139.5, 373.6034)
  line L958 (139.5, 373.6034) -> (139.5, 359.0541)
  line L959 (139.5, 359.0541) -> (126.9, 351.7795)
  line L960 (126.9, 351.7795) -> (114.3, 359.0541)
  line L961 (114.3, 359.0541) -> (114.3, 373.6034)
  line L962 (114.3, 373.6034) -> (126.9, 380.878)
  line L963 (112.8, 405.2999) -> (125.4, 398.0253)
  line L964 (125.4, 398.0253) -> (125.4, 383.476)
  line L965 (125.4, 383.476) -> (112.8, 376.2014)
  line L966 (112.8, 376.2014) -> (100.2, 383.476)
  line L967 (100.2, 383.476) -> (100.2, 398.0253)
  line L968 (100.2, 398.0253) -> (112.8, 405.2999)
  line L969 (98.7, 429.7218) -> (111.3, 422.4472)
  line L970 (111.3, 422.4472) -> (111.3, 407.898)
  line L971 (111.3, 407.898) -> (98.7, 400.6234)
  line L972 (98.7, 400.6234) -> (86.1, 407.898)
  line L973 (86.1, 407.898) -> (86.1, 422.4472)
  line L974 (86.1, 422.4472) -> (98.7, 429.7218)
  line L975 (84.6, 454.1437) -> (97.2, 446.8691)
  line L976 (97.2, 446.8691) -> (97.2, 432.3199)
  line L977 (97.2, 432.3199) -> (84.6, 425.0453)
  line L978 (84.6, 425.0453) -> (72, 432.3199)
  line L979 (72, 432.3199) -> (72, 446.8691)
  line L980 (72, 446.8691) -> (84.6, 454.1437)
  line L981 (70.5, 478.5656) -> (83.1, 471.291)
  line L982 (83.1, 471.291) -> (83.1, 456.7418)
  line L983 (83.1, 456.7418) -> (70.5, 449.4672)
  line L984 (70.5, 449.4672) -> (57.9, 456.7418)
  line L985 (57.9, 456.7418) -> (57.9, 471.291)
  line L986 (57.9, 471.291) -> (70.5, 478.5656)
  line L987 (56.4, 502.9876) -> (69, 495.7129)
  line L988 (69, 495.7129) -> (69, 481.1637)
  line L989 (69, 481.1637) -> (56.4, 473.8891)